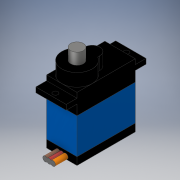
# Autodesk Inventor part: TP-MG92B
Saved by Autodesk Inventor 2017 (Build 210142000, 142)
## iProperties
Created: 2017-08-24
Part Number: TP-MG92B
Material: Generic
Document SubType Name: Modeling
Designer: Alexander Miller
Density: 1 g/cm^3
Appearance: Default
servo_A: 23,000 mm
servo_B: 12,000 mm
servo_C: 30,000 mm
servo_D: 31,500 mm
servo_E: 21,000 mm
servo_F: 2,000 mm
servo_G: 5,000 mm
servo_H: 2,000 mm
servo_I: 15,000 mm
servo_J: 2,000 mm
servo_K: 5,000 mm
servo_L: 1,500 mm
servo_M: 5,000 mm
servo_N: 6,000 mm
servo_O: 34,500 mm
servo_P: 33,000 mm
Author: Alexander Miller
Autodesk Inventor part; units mm, degrees
ref_plane "YZ Plane" through (0, 0, 0) normal (1, 0, 0) x (0, 1, 0)
sketch "Sketch1" plane through (0, 0, 0) normal (0, 1, 0) x (-1, 0, 0)
  line L0 (6, 11.5) -> (-6, 11.5)
  line L1 (-6, 11.5) -> (-6, -11.5)
  line L2 (-6, -11.5) -> (6, -11.5)
  line L3 (6, -11.5) -> (6, 11.5)
  point P0 (0, 0)
  point P1 (6, 0)
  point P2 (0, 11.5)
  dimension "d0" = 23
  dimension "d1" = 12
  constraints: 8 end point, 2 midpoint, 2 parallel, 1 horizontal, 1 horizontal alignment, 1 perpendicular, 1 vertical alignment
  measures "d0" distance of L2.end L0.start
  measures "d1" distance of L1.end L2.end
extrude "Extrusion1" add sketch "Sketch1" along normal blind 25
sketch "Sketch2" plane through (-6, 0, 11.5) normal (0, 0, 1) x (1, 0, 0)
  line L0 (0, 23) -> (12, 23)
  line L1 (12, 23) -> (12, 21)
  line L2 (12, 21) -> (0, 21)
  line L3 (0, 21) -> (0, 23)
  line L4 (0, 0) -> (0, 25) projected
  line L5 (12, 0) -> (12, 25) projected
  line L6 (0, 0) -> (12, 0) projected
  point P0 (6, 0)
  dimension "d4" = 2
  dimension "d5" = 21
  constraints: 8 end point, 2 collinear, 2 parallel, 1 horizontal, 1 perpendicular
  measures "d4" distance between parallel lines of L2 L0
  measures "d5" distance between parallel lines of L6 L2
extrude "Extrusion2" add sketch "Sketch2" along normal blind 4.25 and the other way blind 27.25 contours L0 L1 L2 L3
sketch "Sketch3" plane through (0, 25, 0) normal (0, 1, 0) x (1, 0, 0)
  circle A0 centre (0, -5.5) radius 6
  circle A1 centre (0, 0.5) radius 3
  line L0 (-6, 11.5) -> (-6, -11.5) projected
  line L1 (6, -11.5) -> (6, 11.5) projected
  line L2 (-6, -11.5) -> (6, -11.5) projected
  line L3 (-6, 3.5) -> (6, 3.5) construction
  line L4 (-3, 0.5) -> (-3, -0.3038)
  line L5 (3, 0.5) -> (3, -0.3038)
  point P0 (0, 0)
  point P1 (0, -11.5)
  dimension "d10" = 12
  dimension "d11" = 6
  dimension "d12" = 15
  constraints: 6 end point, 4 point on circle, 4 tangent, 2 centre point, 2 point on line, 2 vertical, 2 vertical alignment, 1 midpoint
  measures "d10" diameter of A0
  measures "d11" diameter of A1
  measures "d12" distance between parallel lines of L2 L3
extrude "Extrusion3" add sketch "Sketch3" along normal blind 5 contours A0 A1 | A0 A1 L5 | A1 A0 | A0 A1 | A0 L4 A1
sketch "Sketch4" plane through (0, 30, 0) normal (0, 1, 0) x (1, 0, 0)
  circle A0 centre (0, -5.5) radius 2.5
  arc A1 (-3, -0.3038) -> (3, -0.3038) centre (0, -5.5) ccw projected
  point P0 (0, 0)
  dimension "d15" = 5
  constraints: 1 centre point, 1 concentric
  measures "d15" diameter of A0
extrude "Extrusion4" add sketch "Sketch4" along normal blind 4.5
sketch "Sketch5" plane through (-6, 0, 11.5) normal (0, 0, 1) x (1, 0, 0)
  line L0 (3.5, 2) -> (8.5, 2)
  line L1 (8.5, 2) -> (8.5, 0)
  line L2 (8.5, 0) -> (3.5, 0)
  line L3 (3.5, 0) -> (3.5, 2)
  line L4 (0, 0) -> (12, 0) projected
  circle A0 centre (4.5, 1) radius 1
  circle A1 centre (7.5, 1) radius 1
  circle A2 centre (6, 1) radius 1
  point P0 (6, 0)
  point P1 (6, 0)
  point P2 (6, 0)
  point P3 (6, 0)
  dimension "d18" = 5
  dimension "d19" = 2
  constraints: 8 end point, 8 tangent, 3 centre point, 3 midpoint, 2 parallel, 1 coincident, 1 collinear, 1 horizontal, 1 perpendicular, 1 vertical alignment
  measures "d18" distance of L0.start L0.end
  measures "d19" distance of L2.end L0.start
extrude "Extrusion5" add sketch "Sketch5" along normal blind 5 contours A0 A2 | A2 A1 A0 | A0 A2 | A1 A2 | A2 A1
ref_plane "Work Plane1" through (0, 3, 0) normal (0, -1, 0) x (1, 0, 0)
ref_plane "Work Plane2" through (0, 17, 0) normal (0, -1, 0) x (1, 0, 0)
split_face "Split1"
split_face "Split2"
sketch "Sketch6" plane through (-6, 23, 11.5) normal (0, 1, 0) x (1, 0, 0)
  circle A0 centre (6, -2.5) radius 1
  line L0 (12, -4.25) -> (0, -4.25) projected
  line L1 (0, 0) -> (12, 0) projected
  point P0 (6, 11.5)
  point P1 (6, -4.25)
  dimension "d24" = 2
  dimension "d25" = 1.5
  constraints: 1 centre point, 1 midpoint, 1 vertical alignment
  measures "d24" diameter of A0
  measures "d25" distance edge to line of A0 L1
extrude "Extrusion6" cut sketch "Sketch6" against normal up to surface (2 mm away)
sketch "Sketch7" plane through (-6, 23, -11.5) normal (0, 1, 0) x (1, 0, 0)
  circle A0 centre (6, 2.5) radius 1
  line L0 (0, 4.25) -> (12, 4.25) projected
  line L1 (12, 0) -> (0, 0) projected
  point P0 (6, -11.5)
  point P1 (6, 4.25)
  dimension "d28" = 2
  dimension "d29" = 1.5
  constraints: 1 centre point, 1 midpoint, 1 vertical alignment
  measures "d28" diameter of A0
  measures "d29" distance edge to line of A0 L1
extrude "Extrusion7" cut sketch "Sketch7" against normal up to surface (2 mm away)
equation "\"d0\" = servo_A"
equation "\"d1\" = servo_B"
equation "\"d2\" = servo_F + servo_E + servo_J"
equation "\"d4\" = servo_F"
equation "\"d5\" = servo_E"
equation "\"d6\" = -0.5 * servo_A + 0.5 * servo_D"
equation "\"d7\" = d6 + servo_A"
equation "\"d10\" = servo_B"
equation "\"d11\" = servo_N"
equation "\"d12\" = servo_I"
equation "\"d13\" = -servo_F + servo_C - servo_E - servo_J"
equation "\"d15\" = servo_G"
equation "\"d16\" = servo_O - servo_C"
equation "\"d18\" = servo_K"
equation "\"d24\" = servo_H"
equation "\"d25\" = servo_L"
equation "\"d28\" = servo_H"
equation "\"d29\" = servo_L"
equation "\"servo_A\" = 23"
equation "\"servo_B\" = 12"
equation "\"servo_C\" = 30"
equation "\"servo_D\" = 31.5"
equation "\"servo_E\" = 21"
equation "\"servo_F\" = 2"
equation "\"servo_G\" = 5"
equation "\"servo_H\" = 2"
equation "\"servo_I\" = 15"
equation "\"servo_J\" = 2"
equation "\"servo_K\" = 5"
equation "\"servo_L\" = 1.5"
equation "\"servo_M\" = 5"
equation "\"servo_N\" = 6"
equation "\"servo_O\" = 34.5"
equation "\"servo_P\" = 33"
body "Solid1"
